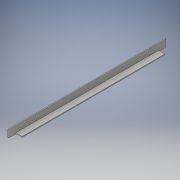
# Autodesk Inventor part: 22 cut 20 L bracket
Saved by Autodesk Inventor 2016 SP2 (Build 200236200, 236)
## iProperties
Created: 2018-01-17
Part Number: 22 cut 20 L bracket
Material: Generic
Document SubType Name: Modeling
Designer: CAD
Density: 1 g/cm^3
Appearance: Default
Author: CAD
Autodesk Inventor part; units mm, degrees
ref_plane "YZ Plane" through (0, 0, 0) normal (1, 0, 0) x (0, 1, 0)
ref_plane "XZ Plane" through (0, 0, 0) normal (0, 1, 0) x (-1, 0, 0)
ref_plane "XY Plane" through (0, 0, 0) normal (0, 0, 1) x (1, 0, 0)
sketch "Sketch1" plane through (0, 0, 0) normal (0, 0, 1) x (1, 0, 0)
  line L0 (0, 0) -> (0, 25.4)
  line L1 (0, 0) -> (25.4, 0)
  line L2 (25.4, 3.175) -> (3.175, 3.175)
  line L3 (3.175, 3.175) -> (3.175, 25.4)
  line L4 (25.4, 3.175) -> (25.4, 0)
  line L5 (0, 25.4) -> (3.175, 25.4)
  dimension "d0" = 25.4
  dimension "d1" = 25.4
  dimension "d2" = 3.175
  constraints: 12 end point, 2 horizontal, 2 vertical, 1 other
  measures "d0" distance of L0.start L0.end
  measures "d1" distance of L0.start L1.end
  measures "d2" distance between parallel lines of L1 L2
extrude "Extrusion1" add sketch "Sketch1" along normal blind 558.8
sketch "Sketch2" plane through (3.175, 3.175, 0) normal (0, 1, 0) x (1, 0, 0)
  line L0 (0, 0) -> (0, -558.8) projected
  line L1 (0, -25.4) -> (22.225, -25.4)
  line L2 (22.225, 0) -> (22.225, -558.8) projected
  line L3 (0, -533.4) -> (22.225, -533.4)
  line L4 (22.225, -558.8) -> (0, -558.8) projected
  line L5 (0, 0) -> (22.225, 0) projected
  line L6 (22.225, -533.4) -> (22.225, -558.8)
  line L7 (0, -558.8) -> (0, -533.4)
  line L8 (-3.175, -558.8) -> (22.225, -558.8) projected
  line L9 (0, -25.4) -> (0, 0)
  line L10 (-3.175, 0) -> (-3.175, -558.8) projected
  line L11 (22.225, 0) -> (-3.175, 0) projected
  line L12 (0, 0) -> (22.225, 0)
  line L13 (22.225, 0) -> (22.225, -25.4)
  line L14 (0, -558.8) -> (22.225, -558.8)
  dimension "d5" = 25.4
  dimension "d6" = 25.4
  constraints: 16 end point, 4 collinear, 4 point on line, 2 perpendicular, 1 horizontal, 1 parallel
  measures "d5" distance between parallel lines of L4 L3
  measures "d6" distance between parallel lines of L5 L1
extrude "Extrusion2" cut sketch "Sketch2" against normal blind 25.4 contours L5 L2 L1 L0 | L3 L2 L4 L0
body "Solid1"
